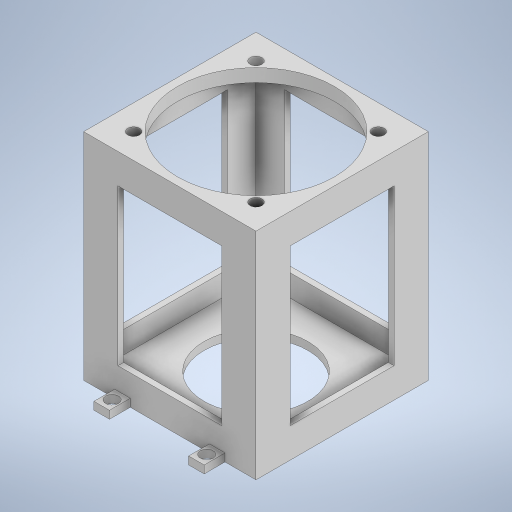
# Autodesk Inventor part: Motor case
Saved by Autodesk Inventor 2023 (Build 270158000, 158)
## iProperties
Created: 2023-02-22
Part Number: Motor case
Material: Generic
Document SubType Name: Modeling
Designer: cheng
Density: 1 g/cm^3
Appearance: Default
Author: cheng
Autodesk Inventor part; units mm, degrees
ref_plane "YZ Plane" through (0, 0, 0) normal (1, 0, 0) x (0, 1, 0)
ref_plane "XZ Plane" through (0, 0, 0) normal (0, 1, 0) x (-1, 0, 0)
ref_plane "XY Plane" through (0, 0, 0) normal (0, 0, 1) x (1, 0, 0)
sketch "Sketch1" plane through (0, 0, 0) normal (0, 1, 0) x (-1, 0, 0)
  line L0 (28.2, -28.2) -> (-28.2, -28.2)
  line L1 (-28.2, -28.2) -> (-28.2, 28.2)
  line L2 (-28.2, 28.2) -> (28.2, 28.2)
  line L3 (28.2, 28.2) -> (28.2, -28.2)
  line L4 (28.2, -28.2) -> (-28.2, 28.2) construction
  line L5 (-28.2, -28.2) -> (28.2, 28.2) construction
  line L6 (33.2, -33.2) -> (-33.2, -33.2)
  line L7 (-33.2, -33.2) -> (-33.2, 33.2)
  line L8 (-33.2, 33.2) -> (33.2, 33.2)
  line L9 (33.2, 33.2) -> (33.2, -33.2)
  line L10 (33.2, -33.2) -> (-33.2, 33.2) construction
  line L11 (-33.2, -33.2) -> (33.2, 33.2) construction
  circle A0 centre (0, 0) radius 20
  line L12 (-21.2465, -33.2) -> (-15.2465, -33.2)
  line L13 (-15.2465, -33.2) -> (-15.2465, -41.2)
  line L14 (-15.2465, -41.2) -> (-21.2465, -41.2)
  line L15 (-21.2465, -41.2) -> (-21.2465, -33.2)
  circle A1 centre (-18.2465, -37.2) radius 2.5
  line L16 (-33.2, 0) -> (33.2, 0) construction
  line L17 (0, -33.2) -> (0, 33.2) construction
  line L18 (-21.2465, 33.2) -> (-15.2465, 33.2)
  line L19 (-15.2465, 33.2) -> (-15.2465, 41.2)
  line L20 (-15.2465, 41.2) -> (-21.2465, 41.2)
  line L21 (-21.2465, 41.2) -> (-21.2465, 33.2)
  circle A2 centre (-18.2465, 37.2) radius 2.5
  line L22 (21.2465, -33.2) -> (15.2465, -33.2)
  line L23 (15.2465, -33.2) -> (15.2465, -41.2)
  line L24 (15.2465, -41.2) -> (21.2465, -41.2)
  line L25 (21.2465, -41.2) -> (21.2465, -33.2)
  circle A3 centre (18.2465, -37.2) radius 2.5
  circle A4 centre (18.2465, 37.2) radius 2.5
  line L26 (15.2465, 33.2) -> (15.2465, 41.2)
  line L27 (15.2465, 41.2) -> (21.2465, 41.2)
  line L28 (21.2465, 41.2) -> (21.2465, 33.2)
  line L29 (21.2465, 33.2) -> (15.2465, 33.2)
  dimension "d0" = 56.4
  dimension "d1" = 5
  dimension "d2" = 5
  dimension "d3" = 40
  dimension "d20" = 6
  dimension "d21" = 5
  dimension "d22" = 3
  dimension "d23" = 4
  dimension "d24" = 8
  constraints: 60 end point, 15 symmetric about line, 8 midpoint, 6 parallel, 5 centre point, 3 horizontal, 3 perpendicular, 2 point on line, 1 coincident, 3 other
  measures "d0" distance between parallel lines of L2 L0
  measures "d1" distance between parallel lines of L7 L1
  measures "d2" distance between parallel lines of L8 L2
  measures "d3" diameter of A0
  measures "d20" distance between parallel lines of L13 L15
  measures "d21" diameter of A1
  measures "d22" distance from line of L15 A1.centre
  measures "d23" distance from line of L14 A1.centre
  measures "d24" distance between parallel lines of L6 L14
extrude "Extrusion1" add sketch "Sketch1" along normal blind 3 contours L0 L1 L2 L3 | L6 L7 L8 L9 | L25 L24 L23 L6 | L8 L26 L27 L28 | L13 L14 L15 L6 | L8 L21 L20 L19
sketch "Sketch2" plane through (0, 3, 0) normal (0, 1, 0) x (1, 0, 0)
  line L0 (-33.2, -33.2) -> (-21.2465, -33.2) projected
  line L1 (33.2, -33.2) -> (33.2, 33.2) projected
  line L2 (33.2, 33.2) -> (21.2465, 33.2) projected
  line L3 (-33.2, 33.2) -> (-33.2, -33.2) projected
  circle A0 centre (0, 0) radius 20 projected
  line L4 (-31, 31) -> (31, 31)
  line L5 (31, 31) -> (31, -31)
  line L6 (31, -31) -> (-31, -31)
  line L7 (-31, -31) -> (-31, 31)
  line L8 (-31, 31) -> (31, -31) construction
  line L9 (31, 31) -> (-31, -31) construction
  line L10 (-21.2465, -33.2) -> (-21.2465, -41.2) projected
  line L11 (-21.2465, -41.2) -> (-15.2465, -41.2) projected
  line L12 (-15.2465, -41.2) -> (-15.2465, -33.2) projected
  line L13 (-15.2465, -33.2) -> (15.2465, -33.2) projected
  line L14 (15.2465, -33.2) -> (15.2465, -41.2) projected
  line L15 (15.2465, -41.2) -> (21.2465, -41.2) projected
  line L16 (21.2465, -41.2) -> (21.2465, -33.2) projected
  line L17 (21.2465, -33.2) -> (33.2, -33.2) projected
  line L18 (21.2465, 33.2) -> (21.2465, 41.2) projected
  line L19 (21.2465, 41.2) -> (15.2465, 41.2) projected
  line L20 (15.2465, 41.2) -> (15.2465, 33.2) projected
  line L21 (15.2465, 33.2) -> (-15.2465, 33.2) projected
  line L22 (-15.2465, 33.2) -> (-15.2465, 41.2) projected
  line L23 (-15.2465, 41.2) -> (-21.2465, 41.2) projected
  line L24 (-21.2465, 41.2) -> (-21.2465, 33.2) projected
  line L25 (-21.2465, 33.2) -> (-33.2, 33.2) projected
  line L26 (33.2, 33.2) -> (21.2465, 33.2) projected
  line L27 (15.2465, 41.2) -> (15.2465, 33.2) projected
  line L28 (33.2, -33.2) -> (33.2, 33.2) projected
  line L29 (33.2, 33.2) -> (-33.2, 33.2)
  line L30 (21.2465, -33.2) -> (33.2, -33.2) projected
  line L31 (33.2, -33.2) -> (-33.2, -33.2)
  dimension "d6" = 62
  dimension "d7" = 62
  constraints: 16 end point, 3 parallel, 2 midpoint, 2 perpendicular, 1 horizontal
  measures "d6" distance between parallel lines of L6 L4
  measures "d7" distance between parallel lines of L7 L5
extrude "Extrusion2" add sketch "Sketch2" along normal blind 75 contours L3 L25 L29 L21 L2 L1 L17 L31 L13 L0
sketch "Sketch3" plane through (0, 78, 0) normal (0, 1, 0) x (1, 0, 0)
  line L0 (33.2, -33.2) -> (33.2, 33.2) projected
  line L1 (33.2, 33.2) -> (-33.2, 33.2) projected
  line L2 (-33.2, 33.2) -> (-33.2, -33.2) projected
  line L3 (-33.2, -33.2) -> (33.2, -33.2) projected
  line L4 (-31, 31) -> (31, 31) projected
  line L5 (31, 31) -> (31, -31) projected
  line L6 (31, -31) -> (-31, -31) projected
  line L7 (-31, -31) -> (-31, 31) projected
  circle A0 centre (0, 0) radius 28.2247 construction
  circle A1 centre (0, 0) radius 30.2247
  point P0 (-30, 3.4699)
  point P1 (-3.4699, 30)
  point P2 (3.4699, 30)
  point P3 (30, 3.4699)
  point P4 (30, -3.4699)
  point P5 (3.4699, -30)
  point P6 (-3.4699, -30)
  point P7 (-30, -3.4699)
  dimension "d11" = 2
  constraints: 2 centre point, 2 coincident
  measures "d11" radial gap between concentric circles of A0 A1
extrude "Extrusion3" add sketch "Sketch3" along normal blind 5 contours L3 L2 L1 L0 | L4 L5 L6 L7
sketch "Sketch4" plane through (0, 83, 0) normal (0, 1, 0) x (1, 0, 0)
  line L0 (33.2, 33.2) -> (-33.2, 33.2) projected
  line L1 (-33.2, 33.2) -> (-33.2, -33.2) projected
  line L2 (-33.2, -33.2) -> (33.2, -33.2) projected
  line L3 (33.2, -33.2) -> (33.2, 33.2) projected
  line L4 (33.2, -33.2) -> (33.2, 33.2) construction
  line L5 (33.2, 0) -> (-33.2, 0) construction
  line L6 (0, 33.2) -> (0, -33.2) construction
  circle A0 centre (23.57, 23.57) radius 2.3
  circle A1 centre (23.57, -23.57) radius 2.3
  circle A2 centre (-23.57, 23.57) radius 2.3
  circle A3 centre (-23.57, -23.57) radius 2.3
  point P0 (0, 0)
  dimension "d14" = 47.14
  dimension "d15" = 4.6
  dimension "d18" = 47.14
  constraints: 4 centre point, 4 end point, 4 midpoint, 3 symmetric about line, 3 other
  measures "d14" distance of A1.centre A0.centre
  measures "d15" diameter of A0
  measures "d18" distance of A3.centre A1.centre
extrude "Extrusion4" cut sketch "Sketch4" against normal blind 10 contours A0 | A1 | A2 | A3
sketch "Sketch5" plane through (33.2, 0, 33.2) normal (1, 0, 0) x (0, 0, -1)
  line L0 (-8, 0) -> (0, 0) projected
  line L1 (-8, 0) -> (0, 0) projected
  line L2 (0, 0) -> (0, 3) projected
  line L3 (-8, 3) -> (0, 3) projected
  line L4 (-8, 0) -> (-8, 3) projected
  line L5 (0, 0) -> (66.4, 0) projected
  line L6 (66.4, 0) -> (66.4, 83) projected
  line L7 (0, 83) -> (66.4, 83) projected
  line L8 (0, 0) -> (0, 83) projected
  line L9 (66.4, 3) -> (74.4, 3) projected
  line L10 (66.4, 0) -> (74.4, 0) projected
  line L11 (66.4, 0) -> (74.4, 0) projected
  line L12 (74.4, 0) -> (74.4, 3) projected
  line L13 (66.4, 3) -> (74.4, 3) projected
  line L14 (66.4, 0) -> (66.4, 3) projected
  line L15 (74.4, 3) -> (66.4, 3) construction
  line L16 (0, 3) -> (66.4, 3) construction
  line L17 (33.2, 0) -> (33.2, 83) construction
  line L18 (0, 0) -> (0, 83) construction
  line L19 (0, 41.5) -> (66.4, 41.5) construction
  line L20 (66.4, 0) -> (66.4, 83) construction
  line L21 (13.2, 71.5) -> (53.2, 71.5)
  line L22 (53.2, 71.5) -> (53.2, 11.5)
  line L23 (53.2, 11.5) -> (13.2, 11.5)
  line L24 (13.2, 11.5) -> (13.2, 71.5)
  line L25 (13.2, 71.5) -> (53.2, 11.5) construction
  line L26 (53.2, 71.5) -> (13.2, 11.5) construction
  point P0 (33.2, 41.5)
  dimension "d27" = 40
  dimension "d28" = 60
  constraints: 18 end point, 6 midpoint, 2 parallel, 1 collinear, 1 horizontal, 1 perpendicular
  measures "d27" distance of L21.start L21.end
  measures "d28" distance between parallel lines of L23 L21
extrude "Extrusion5" cut sketch "Sketch5" against normal through all contours L21 L22 L23 L24
sketch "Sketch6" plane through (15.2465, 0, -33.2) normal (0, 0, -1) x (-1, 0, 0)
  line L0 (-17.9535, 0) -> (-6, 0) projected
  line L1 (-6, 0) -> (-6, 3) projected
  line L2 (0, 3) -> (-6, 3) projected
  line L3 (0, 0) -> (0, 3) projected
  line L4 (0, 0) -> (30.493, 0) projected
  line L5 (30.493, 0) -> (30.493, 3) projected
  line L6 (36.493, 3) -> (30.493, 3) projected
  line L7 (36.493, 0) -> (36.493, 3) projected
  line L8 (36.493, 0) -> (48.4465, 0) projected
  line L9 (48.4465, 0) -> (48.4465, 83) projected
  line L10 (-17.9535, 83) -> (48.4465, 83) projected
  line L11 (-17.9535, 0) -> (-17.9535, 83) projected
  line L12 (-17.9535, 11.5) -> (-17.9535, 71.5) construction
  line L13 (-17.9535, 41.5) -> (48.4465, 41.5) construction
  line L14 (48.4465, 0) -> (48.4465, 83) construction
  line L15 (48.4465, 83) -> (-17.9535, 83) construction
  line L16 (15.2465, 83) -> (15.2465, 0) construction
  line L17 (-4.7535, 71.5) -> (35.2465, 71.5)
  line L18 (35.2465, 71.5) -> (35.2465, 11.5)
  line L19 (35.2465, 11.5) -> (-4.7535, 11.5)
  line L20 (-4.7535, 11.5) -> (-4.7535, 71.5)
  line L21 (-4.7535, 71.5) -> (35.2465, 11.5) construction
  line L22 (35.2465, 71.5) -> (-4.7535, 11.5) construction
  point P0 (15.2465, 41.5)
  dimension "d29" = 40
  dimension "d30" = 60
  constraints: 16 end point, 6 midpoint, 2 parallel, 1 horizontal, 1 perpendicular, 1 vertical
  measures "d29" distance between parallel lines of L18 L20
  measures "d30" distance between parallel lines of L19 L17
extrude "Extrusion6" cut sketch "Sketch6" against normal up to surface (66.4 mm away) contours L17 L18 L19 L20
body "Solid1"
